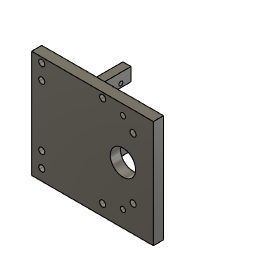
ServoMount v4 (Autodesk Fusion 360 design; units mm, degrees)
Autodesk Fusion 360 part; units mm, degrees
note: some values were not read from the file. Set by a fixed rule: which sketch regions a step uses.
sketch "Sketch1" plane through (0, 0, 0) normal (0, 0, 1) x (1, 0, 0)
  line L0 (0, 0) -> (60, 0)
  line L1 (60, 0) -> (60, 50)
  line L2 (60, 50) -> (0, 50)
  line L3 (0, 50) -> (0, 0)
  line L4 (0, 50) -> (5, 50)
  line L5 (5, 50) -> (5, 47.5)
  line L6 (5, 47.5) -> (0, 47.5)
  line L7 (0, 47.5) -> (0, 50)
  line L8 (0, 0) -> (5, 0)
  line L9 (5, 0) -> (5, 2.5)
  line L10 (5, 2.5) -> (0, 2.5)
  line L11 (0, 2.5) -> (0, 0)
  circle A0 centre (5, 2.5) radius 1.5
  circle A1 centre (5, 47.5) radius 1.5
  line L12 (5, 47.5) -> (35, 47.5)
  line L13 (5, 2.5) -> (35, 2.5)
  line L14 (5, 50) -> (5, 40)
  line L15 (5, 0) -> (5, 10)
  line L16 (5, 40) -> (50, 40)
  line L17 (5, 10) -> (50, 10)
  line L18 (60, 50) -> (60, 45)
  line L19 (60, 45) -> (45, 45)
  circle A2 centre (45, 45) radius 1.25
  line L20 (60, 0) -> (60, 5)
  line L21 (60, 5) -> (45, 5)
  circle A3 centre (45, 5) radius 1.25
  line L22 (60, 0) -> (60, 25)
  line L23 (60, 25) -> (45, 25)
  circle A4 centre (45, 25) radius 6.25
  circle A5 centre (50, 40) radius 1.5
  circle A6 centre (5, 10) radius 1.5
  circle A7 centre (50, 10) radius 1.5
  circle A8 centre (35, 47.5) radius 1.5
  circle A9 centre (35, 2.5) radius 1.5
  dimension "d1" = 60
  dimension "d2" = 50
  dimension "d3" = 5
  dimension "d4" = 2.5
  dimension "d5" = 5
  dimension "d6" = 2.5
  dimension "d7" = 3
  dimension "d8" = 3
  dimension "d9" = 30
  dimension "d10" = 30
  dimension "d11" = 10
  dimension "d12" = 10
  dimension "d13" = 45
  dimension "d14" = 45
  dimension "d15" = 15
  dimension "d16" = 2.5
  dimension "d17" = 5
  dimension "d18" = 15
  dimension "d19" = 2.5
  dimension "d20" = 15
  dimension "d21" = 12.5
  dimension "d22" = 3
  dimension "d23" = 3
  dimension "d24" = 3
  dimension "d25" = 3
  dimension "d26" = 3
  constraint horizontal L0
  constraint vertical L1
  constraint horizontal L2
  constraint vertical L3
  constraint coincident L0.start L3.end
  constraint horizontal L4
  constraint vertical L5
  constraint horizontal L6
  constraint vertical L7
  constraint horizontal L8
  constraint vertical L9
  constraint horizontal L10
  constraint vertical L11
  constraint coincident L9.end L10.start
  constraint coincident L5.end L6.start
  constraint perpendicular L5 L12
  constraint perpendicular L9 L13
  constraint perpendicular L4 L14
  constraint perpendicular L0 L15
  constraint perpendicular L14 L16
  constraint perpendicular L15 L17
  constraint coincident L1 L18.end
  constraint perpendicular L18 L19
  constraint coincident L19.end A2.centre
  constraint perpendicular L0 L20
  constraint perpendicular L20 L21
  constraint coincident L21.end A3.centre
  constraint midpoint L1 L22.end
  constraint perpendicular L22 L23
  constraint coincident L23.end A4.centre
  constraint coincident L16.end A5.centre
  constraint coincident L15.end L17.start
  constraint coincident L17.end A7.centre
  constraint coincident L12.end A8.centre
  constraint coincident L13.end A9.centre
  measures "d1" distance of L0.start L0.end
  measures "d2" distance of L0.start L2.end
  measures "d3" distance of L2.end L4.end
  measures "d4" distance of L2.end L6.end
  measures "d5" distance of L0.start L8.end
  measures "d6" distance of L0.start L10.end
  measures "d7" diameter of A0
  measures "d8" diameter of A1
  measures "d9" distance of L5.end L12.end
  measures "d10" distance of L9.end L13.end
  measures "d11" distance of L4.end L14.end
  measures "d12" distance of L8.end L15.end
  measures "d13" distance of L14.end L16.end
  measures "d14" distance of L15.end L17.end
  measures "d15" distance of L18.end L19.end
  measures "d16" diameter of A2
  measures "d17" distance of L0.end L20.end
  measures "d18" distance of L20.end L21.end
  measures "d19" diameter of A3
  measures "d20" distance of L22.end L23.end
  measures "d21" diameter of A4
  measures "d22" diameter of A5
  measures "d23" diameter of A6
  measures "d24" diameter of A7
  measures "d25" diameter of A8
  measures "d26" diameter of A9
extrude "Extrude1" add sketch "Sketch1" along normal blind 5 contours L0 L3 L8 L9 L10 L11 A0 L15 | L0 L1 L2 L3 L5 L6 L9 L10 A0 A1 L14 L15 L18 L20 L22 | L2 L3 L4 L5 L6 L7 A1 L14
sketch "Sketch2" plane through (0, 0, 5) normal (0, 0, 1) x (1, 0, 0)
  circle A0 centre (5, 2.5) radius 1.5
  circle A1 centre (5, 10) radius 1.5
  circle A2 centre (35, 2.5) radius 1.5
  circle A3 centre (45, 45) radius 1.25
  circle A4 centre (35, 47.5) radius 1.5
  circle A5 centre (50, 40) radius 1.5
  circle A6 centre (50, 10) radius 1.5
  circle A7 centre (45, 5) radius 1.25
  circle A8 centre (45, 25) radius 6.25
  circle A9 centre (5, 47.5) radius 1.5
  line L0 (0, 50) -> (0, 0)
  line L1 (0, 0) -> (60, 0)
  line L2 (60, 0) -> (60, 50)
  line L3 (60, 50) -> (0, 50)
  line L4 (50, 40) -> (5, 40)
  circle A10 centre (5, 40) radius 1.5
  dimension "d29" = 45
  dimension "d30" = 3
  constraint coincident A5.centre L4.start
  constraint horizontal L4
  constraint coincident L4.end A10.centre
  measures "d29" distance of A5.centre L4.end
  measures "d30" diameter of A10
extrude "Extrude2" cut sketch "Sketch2" against normal blind 5 contours A10
sketch "Sketch3" plane through (0, 0, 0) normal (0, 0, -1) x (-1, 0, 0)
  circle A0 centre (-5, 40) radius 1.5
  circle A1 centre (-5, 2.5) radius 1.5
  circle A2 centre (-5, 10) radius 1.5
  circle A3 centre (-35, 2.5) radius 1.5
  circle A4 centre (-45, 45) radius 1.25
  circle A5 centre (-35, 47.5) radius 1.5
  circle A6 centre (-50, 40) radius 1.5
  circle A7 centre (-50, 10) radius 1.5
  circle A8 centre (-45, 5) radius 1.25
  circle A9 centre (-45, 25) radius 6.25
  circle A10 centre (-5, 47.5) radius 1.5
  line L0 (0, 0) -> (0, 50)
  line L1 (0, 50) -> (-60, 50)
  line L2 (-60, 50) -> (-60, 0)
  line L3 (-60, 0) -> (0, 0)
  line L4 (0, 0) -> (-10, 0)
  line L5 (-10, 0) -> (-14, 0)
  line L6 (-14, 0) -> (-14, 30)
  line L7 (-14, 30) -> (-10, 30)
  line L8 (-10, 30) -> (-10, 0)
  dimension "d33" = 10
  dimension "d34" = 4
  dimension "d35" = 30
  constraint coincident L0.start L3.end
  constraint perpendicular L0 L4
  constraint horizontal L5
  constraint vertical L6
  constraint horizontal L7
  constraint vertical L8
  measures "d33" distance of L0.start L4.end
  measures "d34" distance of L4.end L5.end
  measures "d35" distance of L4.end L7.end
extrude "Extrude3" add sketch "Sketch3" along normal blind 20 contours L3 L5 L6 L7 L8
sketch "Sketch4" plane through (0, 0, -20) normal (0, 0, -1) x (-1, 0, 0)
  line L0 (-10, 30) -> (-14, 30)
  line L1 (-14, 30) -> (-14, 0)
  line L2 (-14, 0) -> (-10, 0)
  line L3 (-10, 0) -> (-10, 30)
  line L4 (-14, 30) -> (-10, 30)
  line L5 (-10, 30) -> (-10, 26.5)
  line L6 (-10, 26.5) -> (-14, 26.5)
  line L7 (-14, 26.5) -> (-14, 30)
  line L8 (-10, 0) -> (-14, 0)
  line L9 (-14, 0) -> (-14, 3.5)
  line L10 (-14, 3.5) -> (-10, 3.5)
  line L11 (-10, 3.5) -> (-10, 0)
  dimension "d38" = 3.5
  dimension "d39" = 3.5
  constraint horizontal L4
  constraint vertical L5
  constraint horizontal L6
  constraint vertical L7
  constraint coincident L0.end L1.start
  constraint horizontal L8
  constraint vertical L9
  constraint horizontal L10
  constraint vertical L11
  constraint coincident L2.end L3.start
  measures "d38" distance of L0.end L6.end
  measures "d39" distance of L2.end L10.end
extrude "Extrude4" add sketch "Sketch4" along normal blind 10 contours L0 L1 L3 L4 L5 L6 L7 | L1 L2 L3 L8 L9 L10 L11
sketch "Sketch5" plane through (10, 0, 0) normal (-1, 0, 0) x (0, 0, 1)
  line L0 (0, 0) -> (0, 30)
  line L1 (0, 30) -> (-30, 30)
  line L2 (-30, 30) -> (-30, 26.5)
  line L3 (-30, 26.5) -> (-20, 26.5)
  line L4 (-20, 26.5) -> (-20, 3.5)
  line L5 (-20, 3.5) -> (-30, 3.5)
  line L6 (-30, 3.5) -> (-30, 0)
  line L7 (-30, 0) -> (0, 0)
  line L8 (-30, 30) -> (-30, 28.25)
  line L9 (-30, 28.25) -> (-25, 28.25)
  line L10 (-30, 0) -> (-30, 1.75)
  line L11 (-30, 1.75) -> (-25, 1.75)
  circle A0 centre (-25, 28.25) radius 1
  circle A1 centre (-25, 1.75) radius 1
  dimension "d42" = 5
  dimension "d43" = 2
  dimension "d44" = 2
  constraint coincident L1.end L2.start
  constraint midpoint L2 L8.end
  constraint perpendicular L8 L9
  constraint coincident L6.end L7.start
  constraint midpoint L6 L10.end
  constraint perpendicular L10 L11
  constraint coincident L9.end A0.centre
  constraint coincident L11.end A1.centre
  measures "d42" distance of L8.end L9.end
  measures "d43" diameter of A0
  measures "d44" diameter of A1
extrude "Extrude5" cut sketch "Sketch5" against normal blind 4 contours A0 | A1
sketch "Sketch6" plane through (0, 0, 0) normal (0, 0, -1) x (-1, 0, 0)
  line L0 (-14, 0) -> (-14, 30)
  line L1 (-14, 30) -> (-10, 30)
  line L2 (-10, 30) -> (-10, 0)
  line L3 (-10, 0) -> (0, 0)
  line L4 (0, 0) -> (0, 50)
  line L5 (0, 50) -> (-60, 50)
  line L6 (-60, 50) -> (-60, 0)
  line L7 (-60, 0) -> (-14, 0)
  circle A0 centre (-5, 47.5) radius 1.5
  circle A1 centre (-45, 25) radius 6.25
  circle A2 centre (-45, 5) radius 1.25
  circle A3 centre (-50, 10) radius 1.5
  circle A4 centre (-50, 40) radius 1.5
  circle A5 centre (-35, 47.5) radius 1.5
  circle A6 centre (-45, 45) radius 1.25
  circle A7 centre (-35, 2.5) radius 1.5
  circle A8 centre (-5, 10) radius 1.5
  circle A9 centre (-5, 2.5) radius 1.5
  circle A10 centre (-5, 40) radius 1.5
  line L8 (-10, 0) -> (-10, 5)
  line L9 (-10, 30) -> (-10, 25)
  line L10 (-10, 5) -> (0, 5)
  line L11 (0, 5) -> (0, 8)
  line L12 (0, 8) -> (-10, 8)
  line L13 (-10, 8) -> (-10, 5)
  line L14 (-10, 25) -> (0, 25)
  line L15 (0, 25) -> (0, 22)
  line L16 (0, 22) -> (-10, 22)
  line L17 (-10, 22) -> (-10, 25)
  dimension "d47" = 5
  dimension "d48" = 3
  constraint coincident L2.end L3.start
  constraint coincident L2 L8.end
  constraint perpendicular L3 L8
  constraint coincident L1.end L2.start
  constraint perpendicular L1 L9
  constraint horizontal L10
  constraint vertical L11
  constraint horizontal L12
  constraint vertical L13
  constraint coincident L4 L11.end
  constraint horizontal L14
  constraint vertical L15
  constraint horizontal L16
  constraint vertical L17
  measures "d47" distance of L1.end L9.end
  measures "d48" distance of L9.end L16.end
extrude "Extrude6" add sketch "Sketch6" along normal blind 20 contours L2 L4 L14 L15 L16 L17 | L2 L4 L10 L11 L12 L13
chamfer "Chamfer1" distance 10 distance2 20 2 edges at (0, 23.5, -20) (0, 6.5, -20) measured on face at (12.6667, 12.6667, -20) measured on face at (12.6667, 12.6667, -20)
extrude "Extrude7" add 1 faces at (12.6667, 30, -10) along direction (0, 1, 0) blind 3
extrude "Extrude8" add 1 faces at (24.6667, 0, 3.3333) along direction (0, -1, 0) blind 3
